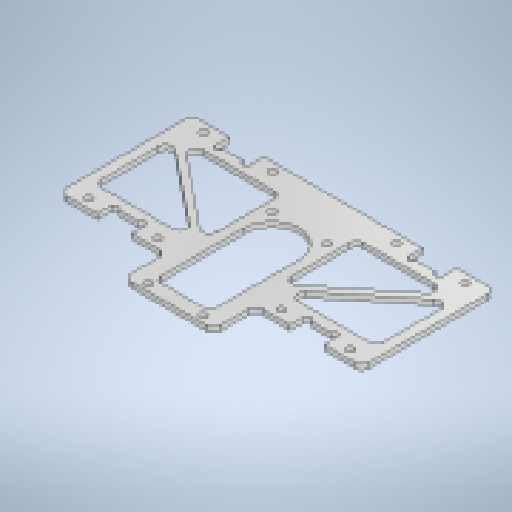
# Autodesk Inventor part: KSHI
Saved by Autodesk Inventor 2025.1 (Build 291241000, 241)
## iProperties
Created: 2023-03-27
Part Number: KSHI
Material: アルミニウム 2014-T4
Document SubType Name: モデリング
Designer: right
Density: 2.8 g/cm^3
Appearance: サテン
Mass: 7.22496 g
Surface Area: 46.2924 cm^2
Volume: 2.58034 cm^3
Sheet Metal Rule: Default
Author: right
Autodesk Inventor part; units mm, degrees
ref_plane "YZ Plane" through (0, 0, 0) normal (1, 0, 0) x (0, 1, 0)
ref_plane "XZ Plane" through (0, 0, 0) normal (0, 1, 0) x (-1, 0, 0)
ref_plane "XY Plane" through (0, 0, 0) normal (0, 0, 1) x (1, 0, 0)
sketch "スケッチ1" plane through (0, 0, 0) normal (0, 1, 0) x (-1, 0, 0)
  line L0 (8, 18) -> (-8, 18) construction
  line L1 (-8, 18) -> (-8, -18) construction
  line L2 (-8, -18) -> (8, -18) construction
  line L3 (8, -18) -> (8, 18) construction
  line L4 (8, 18) -> (-8, -18) construction
  line L5 (-8, 18) -> (8, -18) construction
  circle A0 centre (8, -18) radius 1.1
  circle A1 centre (-8, -18) radius 1.1
  circle A2 centre (8, 18) radius 1.1
  circle A3 centre (-8, 18) radius 1.1
  line L6 (13, 20) -> (-13, 20)
  line L7 (-13, 20) -> (-13, -20)
  line L8 (-13, -20) -> (13, -20)
  line L9 (13, -20) -> (13, 20)
  line L10 (13, 20) -> (-13, -20) construction
  line L11 (-13, 20) -> (13, -20) construction
  line L12 (8, -10) -> (-8, -10)
  line L13 (-8, -10) -> (-8, 16)
  line L14 (-8, 16) -> (8, 16)
  line L15 (8, 16) -> (8, -10)
  circle A4 centre (0, -10) radius 8
  point P0 (0, 0)
  dimension "d0" = 2.2
  dimension "d1" = 16
  dimension "d2" = 36
  dimension "d5" = 16
  dimension "d8" = 36
  dimension "d11" = 2
  dimension "d12" = 5
  dimension "d15" = 2
  dimension "d16" = 10
  constraints: 32 end point, 6 parallel, 5 midpoint, 4 centre point, 4 horizontal, 3 perpendicular, 2 vertical alignment, 1 coincident, 1 vertical, 9 other
  measures "d0" diameter of A0
  measures "d1" distance of L1.end L2.end
  measures "d2" distance of L0.end L1.end
  measures "d5" distance of A0.centre A1.centre
  measures "d8" distance of A0.centre A2.centre
  measures "d11" distance from line of L8 A1.centre
  measures "d12" distance from line of L7 A3.centre
  measures "d15" distance between parallel lines of L0 L14
  measures "d16" distance between parallel lines of L8 L12
extrude "押し出し1" add sketch "スケッチ1" along normal blind 1.5
fillet "フィレット1" radius 2 2 edges at (8, 0.75, 16) (-8, 0.75, 16)
sketch "スケッチ2" plane through (0, 1.5, 0) normal (0, 1, 0) x (1, 0, 0)
  line L0 (-44, -7.75) -> (44, -7.75)
  line L1 (44, -7.75) -> (44, 30.75)
  line L2 (44, 30.75) -> (-44, 30.75)
  line L3 (-44, 30.75) -> (-44, -7.75)
  line L4 (-44, -7.75) -> (44, 30.75) construction
  line L5 (44, -7.75) -> (-44, 30.75) construction
  line L6 (13, 20) -> (-13, 20) projected
  line L7 (-13, 20) -> (-13, -20) projected
  line L8 (-8, -14) -> (-8, 10) projected
  line L9 (8, 10) -> (8, -14) projected
  line L10 (13, -20) -> (13, 20) projected
  line L11 (13, 20) -> (-13, 20) projected
  line L12 (-13, 20) -> (-13, -20) projected
  line L13 (-13, -20) -> (13, -20) projected
  circle A0 centre (-8, -18) radius 1.1 projected
  circle A1 centre (8, -18) radius 1.1 projected
  circle A2 centre (8, 18) radius 1.1 projected
  circle A3 centre (-8, 18) radius 1.1 projected
  line L14 (-8, -14) -> (-8, 10) projected
  arc A4 (8, 10) -> (-8, 10) centre (0, 10) ccw projected
  line L15 (8, 10) -> (8, -14) projected
  arc A5 (6, -16) -> (8, -14) centre (6, -14) ccw projected
  line L16 (6, -16) -> (-6, -16) projected
  arc A6 (-8, -14) -> (-6, -16) centre (-6, -14) ccw projected
  line L17 (33, 26.75) -> (23, 26.75)
  line L18 (23, 26.75) -> (23, 29.75)
  line L19 (23, 29.75) -> (33, 29.75)
  line L20 (33, 29.75) -> (33, 26.75)
  circle A7 centre (38, 28.25) radius 1.1
  line L21 (28, 26.75) -> (28, 29.75) construction
  circle A8 centre (18, 28.25) radius 1.1
  line L22 (44, 11.5) -> (-44, 11.5) construction
  line L23 (33, -3.75) -> (23, -3.75)
  line L24 (23, -3.75) -> (23, -6.75)
  line L25 (23, -6.75) -> (33, -6.75)
  line L26 (33, -6.75) -> (33, -3.75)
  circle A9 centre (38, -5.25) radius 1.1
  line L27 (28, -3.75) -> (28, -6.75) construction
  circle A10 centre (18, -5.25) radius 1.1
  line L28 (0, 30.75) -> (0, -7.75) construction
  line L29 (-33, 26.75) -> (-23, 26.75)
  line L30 (-23, 26.75) -> (-23, 29.75)
  line L31 (-23, 29.75) -> (-33, 29.75)
  line L32 (-33, 29.75) -> (-33, 26.75)
  circle A11 centre (-38, 28.25) radius 1.1
  line L33 (-28, 26.75) -> (-28, 29.75) construction
  circle A12 centre (-18, 28.25) radius 1.1
  circle A13 centre (-18, -5.25) radius 1.1
  line L34 (-23, -3.75) -> (-23, -6.75)
  line L35 (-28, -3.75) -> (-28, -6.75) construction
  line L36 (-33, -3.75) -> (-23, -3.75)
  line L37 (-23, -6.75) -> (-33, -6.75)
  line L38 (-33, -6.75) -> (-33, -3.75)
  circle A14 centre (-38, -5.25) radius 1.1
  circle A15 centre (-31.9, -6.75) radius 1.1
  circle A16 centre (-24.1, -6.75) radius 1.1
  line L39 (-33, -5.25) -> (-28, -5.25) construction
  circle A17 centre (-31.9, -3.75) radius 1.1
  circle A18 centre (-24.1, -3.75) radius 1.1
  circle A19 centre (-31.9, 29.75) radius 1.1
  circle A20 centre (-24.1, 29.75) radius 1.1
  circle A21 centre (-31.9, 26.75) radius 1.1
  circle A22 centre (-24.1, 26.75) radius 1.1
  circle A23 centre (31.9, -6.75) radius 1.1
  circle A24 centre (24.1, -6.75) radius 1.1
  circle A25 centre (31.9, -3.75) radius 1.1
  circle A26 centre (24.1, -3.75) radius 1.1
  circle A27 centre (31.9, 29.75) radius 1.1
  circle A28 centre (31.9, 26.75) radius 1.1
  circle A29 centre (24.1, 26.75) radius 1.1
  circle A30 centre (24.1, 29.75) radius 1.1
  line L40 (33, 29.75) -> (33, 30.75)
  line L41 (23, 29.75) -> (23, 30.75)
  line L42 (-33, 29.75) -> (-33, 30.75)
  line L43 (-23, 29.75) -> (-23, 30.75)
  line L44 (33, -6.75) -> (33, -7.75)
  line L45 (23, -6.75) -> (23, -7.75)
  line L46 (-33, -6.75) -> (-33, -7.75)
  line L47 (-23, -6.75) -> (-23, -7.75)
  point P0 (0, 0)
  point P1 (0, 11.5)
  point P2 (-13, -7.75)
  point P3 (13, -7.75)
  point P4 (33, 28.25)
  point P5 (33, -5.25)
  point P6 (-13, 20)
  point P7 (-13, 20)
  point P8 (-33, 28.25)
  point P9 (33, -3.75)
  point P10 (33, -6.75)
  point P11 (30.8, -6.75)
  point P12 (25.2, -6.75)
  point P13 (23, -6.75)
  point P14 (23, -3.75)
  point P15 (23, -3.75)
  point P16 (-23, 29.75)
  point P17 (-23, 26.75)
  point P18 (-25.2, 26.75)
  point P19 (-30.8, 26.75)
  point P20 (-33, 26.75)
  point P21 (-33, 29.75)
  point P22 (-23, -3.75)
  point P23 (-23, -6.75)
  point P24 (-25.2, -6.75)
  point P25 (-30.8, -6.75)
  point P26 (-33, -3.75)
  point P27 (33, 29.75)
  point P28 (33, 26.75)
  point P29 (30.8, 26.75)
  point P30 (25.2, 26.75)
  point P31 (23, 26.75)
  point P32 (23, 29.75)
  point P33 (23, 29.75)
  point P34 (24.2, -6.75)
  point P35 (-29.8, 26.75)
  point P36 (24.2, 26.75)
  point P37 (27.2, -3.75)
  point P38 (23, -6.75)
  point P39 (30.8, -3.75)
  point P40 (-25.2, 29.75)
  point P41 (-32.8, 29.75)
  point P42 (27.2, 29.75)
  point P43 (30.8, 29.75)
  point P44 (23, 26.75)
  point P45 (-32.8, -3.75)
  point P46 (26.2, -3.75)
  point P47 (-31.8, 29.75)
  point P48 (-31.8, -3.75)
  point P49 (-25.2, -3.75)
  point P50 (26.2, 29.75)
  point P51 (25.2, -3.75)
  point P52 (-30.8, 29.75)
  point P53 (-30.8, -3.75)
  point P54 (25.2, 29.75)
  point P55 (32.3583, 30.75)
  point P56 (23.6417, 30.75)
  point P57 (-23.6417, 30.75)
  point P58 (-32.3583, 30.75)
  point P59 (-32.3583, -7.75)
  point P60 (-23.6417, -7.75)
  point P61 (23.6417, -7.75)
  point P62 (32.3583, -7.75)
  dimension "d30" = 2.2
  dimension "d19" = 31
  dimension "d22" = 10
  dimension "d23" = 3
  dimension "d25" = 2.2
  dimension "d26" = 5
  dimension "d27" = 6
  dimension "d29" = 1
  dimension "d31" = 18.25
  constraints: 74 end point, 52 symmetric about line, 23 centre point, 10 midpoint, 4 parallel, 3 point on line, 2 horizontal, 2 perpendicular, 1 horizontal alignment, 25 other
  measures "d19" distance between parallel lines of L7 L3
  measures "d22" distance of L18.end L19.end
  measures "d23" distance of L17.end L18.end
  measures "d25" diameter of A7
  measures "d26" distance of point (33, 28.25) A7.centre
  measures "d27" distance from line of L1 A7.centre
  measures "d29" distance between parallel lines of L2 L19
  measures "d31" distance between parallel lines of L22 L19
extrude "押し出し3" add sketch "スケッチ2" against normal blind 1.5 contours L3 L2 L42 L32 A21 L29 A22 L30 L43 L41 L18 A29 L17 A28 L20 L40 L1 L0 L44 L26 A25 L23 A26 L24 L45 L10 L6 L7 L47 L34 A18 L36 A17 L38 L46
fillet "フィレット2" radius 2 8 edges at (44, 0.75, -30.75) (44, 0.75, 7.75) (13, 0.75, 7.75) (13, 0.75, 20) (-13, 0.75, 20) (-13, 0.75, 7.75) (-44, 0.75, 7.75) (-44, 0.75, -30.75)
sketch "スケッチ4" plane through (0, 1.5, 0) normal (0, 1, 0) x (1, 0, 0)
  line L0 (41, 23.65) -> (11, 23.65)
  line L1 (11, 23.65) -> (11, -0.65)
  line L2 (11, -0.65) -> (41, -0.65)
  line L3 (41, -0.65) -> (41, 23.65)
  arc A0 (30.8, 26.75) -> (33, 26.75) centre (31.9, 26.75) ccw projected
  line L4 (44, -5.75) -> (44, 28.75) projected
  arc A1 (33, -3.75) -> (30.8, -3.75) centre (31.9, -3.75) ccw projected
  line L5 (-11, -20) -> (11, -20) construction
  line L6 (0, -20) -> (0, 21) construction
  line L7 (-41, 23.65) -> (-11, 23.65)
  line L8 (-11, 23.65) -> (-11, -0.65)
  line L9 (-11, -0.65) -> (-41, -0.65)
  line L10 (-41, -0.65) -> (-41, 23.65)
  line L11 (-44, -5.75) -> (-44, 28.75)
  line L12 (11, -0.65) -> (41, 23.65) construction
  line L13 (44, 24.7931) -> (12.5888, -0.65)
  line L14 (39.4112, 23.65) -> (11, 0.6369)
  line L15 (-44, 24.7931) -> (-12.5888, -0.65)
  line L16 (-39.4112, 23.65) -> (-11, 0.6369)
  line L17 (8, 10) -> (8, -14) projected
  point P0 (0, 0)
  point P1 (31.9, 25.65)
  point P2 (41, 11.5)
  point P3 (31.9, -2.65)
  point P4 (-41, 11.5)
  point P5 (-15, 23)
  point P6 (41, 22.3631)
  point P7 (39.7412, 23.9172)
  point P8 (11.3299, 0.9041)
  point P9 (-11.3299, 0.9041)
  point P10 (17, 0.7731)
  point P11 (-12.5888, -0.65)
  point P12 (-41, 22.3631)
  point P13 (-39.4112, 23.65)
  point P14 (-17, 0.7731)
  dimension "d39" = 2
  dimension "d40" = 3
  dimension "d41" = 2
  dimension "d43" = 1
  dimension "d48" = 3
  constraints: 30 end point, 13 symmetric about line, 10 point on line, 3 parallel, 2 midpoint, 2 point on circle, 1 horizontal, 1 perpendicular
  measures "d39" distance from line of point (31.9, 25.65) L0
  measures "d40" distance from line of L4 point (41, 11.5)
  measures "d41" distance from line of point (31.9, -2.65) L2
  measures "d43" distance between parallel lines of L12 L13
  measures "d48" distance between parallel lines of L17 L1
extrude "押し出し5" cut sketch "スケッチ4" against normal blind 1.5 contours L14 L1 L0 | L3 L2 L13 | L7 L8 L16 | L15 L9 L10
fillet "フィレット3" radius 2 12 edges at (-39.4112, 0.75, -23.65) (-41, 0.75, -22.3631) (-11, 0.75, -23.65) (-12.5888, 0.75, 0.65) (-41, 0.75, 0.65) (41, 0.75, 0.65) (39.4112, 0.75, -23.65) (41, 0.75, -22.3631) (11, 0.75, -23.65) (12.5888, 0.75, 0.65) (-11, 0.75, -0.6369) (11, 0.75, -0.6369)
equation "\"d5\" = d1"
equation "\"d8\" = d2"
